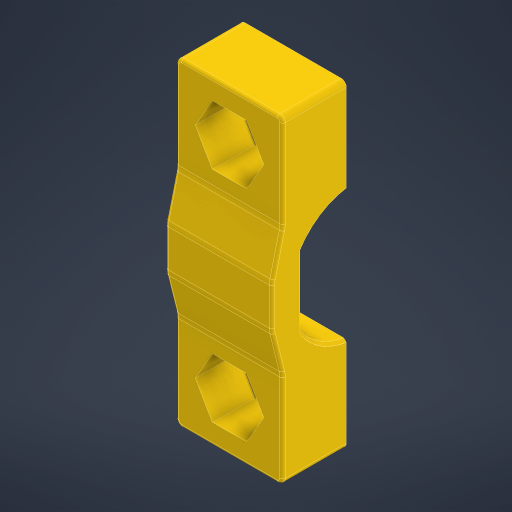
# Autodesk Inventor part: motor_C_clamp_nutt_motor_otoceny
Saved by Autodesk Inventor 2024 (Build 280153000, 153)
## iProperties
Created: 2023-08-14
Part Number: motor_C_clamp_nutt_motor_otoceny
Material: Všeobecné
Document SubType Name: Modeling
Designer: jaryj
Density: 1 g/cm^3
Appearance: Výchozí
Author: jaryj
Autodesk Inventor part; units mm, degrees
ref_plane "YZ Plane" through (0, 0, 0) normal (1, 0, 0) x (0, 1, 0)
ref_plane "XZ Plane" through (0, 0, 0) normal (0, 1, 0) x (-1, 0, 0)
ref_plane "XY Plane" through (0, 0, 0) normal (0, 0, 1) x (1, 0, 0)
sketch "Náčrt1" plane through (0, 0, 0) normal (0, 0, 1) x (1, 0, 0)
  line L0 (-5, 15) -> (5, 15)
  line L1 (5, 15) -> (5, -15)
  line L2 (5, -15) -> (-5, -15)
  line L3 (-5, -15) -> (-5, 15)
  line L4 (-5, 15) -> (5, -15) construction
  line L5 (5, 15) -> (-5, -15) construction
  circle A0 centre (0, 10.3125) radius 1.6
  circle A1 centre (0, -10.3125) radius 1.6
  line L6 (-5, 0) -> (5, 0)
  line L7 (0, 10.3125) -> (0, 15) construction
  line L8 (0, -10.3125) -> (0, -15) construction
  point P0 (0, 0)
  dimension "d0" = 30
  dimension "d1" = 10
  dimension "d2" = 3.2
  dimension "d42" = 20.625
  constraints: 18 end point, 6 midpoint, 2 centre point, 2 parallel, 2 vertical alignment, 1 equal radius, 1 horizontal, 1 perpendicular, 1 vertical, 1 other
  measures "d0" distance of L2.end L0.start
  measures "d1" distance of L0.start L0.end
  measures "d2" diameter of A0
  measures "d42" distance of L8.start L7.start
extrude "Vysunutí1" add sketch "Náčrt1" along normal blind 10
sketch "Náčrt2" plane through (5, -15, 0) normal (1, 0, 0) x (0, 0, -1)
  line L0 (0, 0) -> (0, 30) projected
  line L1 (0, 30) -> (-10, 30) projected
  line L2 (0, 0) -> (-10, 0) projected
  line L3 (-7, 0) -> (-7, 9.0003)
  line L4 (-7, 9.0003) -> (-8, 13)
  line L5 (-8, 17) -> (-7, 20.9997)
  line L6 (-7, 20.9997) -> (-7, 30)
  line L7 (-8, 13) -> (-8, 17)
  line L8 (-10, 0) -> (-10, 30) projected
  line L9 (-5, 11.6835) -> (-5, 18.3165)
  arc A0 (-5, 11.6835) -> (0, 9.0001) centre (0, 15) ccw
  arc A1 (0, 20.9999) -> (-5, 18.3165) centre (0, 15) ccw
  arc A2 (-5.125, 11.646) -> (0, 8.8751) centre (0, 15) ccw
  line L10 (-5.125, 11.646) -> (-5.125, 18.354)
  arc A3 (0, 21.1249) -> (-5.125, 18.354) centre (0, 15) ccw
  arc A4 (-7.5, 11.0001) -> (0, 6.5001) centre (0, 15) ccw construction
  line L11 (-7.5, 11.0001) -> (-7.5, 18.9999) construction
  arc A5 (0, 23.4999) -> (-7.5, 18.9999) centre (0, 15) ccw construction
  point P0 (0, 15)
  point P1 (0, 15)
  point P2 (0, 15)
  point P3 (-8, 15)
  point P4 (-10, 15)
  point P5 (-5, 15)
  point P6 (0, 8.8751)
  dimension "d17" = 3
  dimension "d18" = 3
  dimension "d19" = 2
  dimension "d47" = 6.633
  dimension "d49" = 5
  dimension "d51" = 5.9999
  dimension "d52" = 0.125
  dimension "d53" = 2.5
  dimension "d54" = 4
  constraints: 16 end point, 12 point on circle, 6 centre point, 5 midpoint, 2 coincident, 2 point on line, 1 equal length, 1 horizontal alignment, 1 perpendicular, 1 vertical, 11 other
  measures "d17" distance between parallel lines of L8 L3
  measures "d18" distance between parallel lines of L8 L6
  measures "d19" distance between parallel lines of L8 L7
  measures "d47" distance of L9.start L9.end
  measures "d49" distance of the line from the sketch origin of L9
  measures "d51" radius of A0
  measures "d52" radial gap between concentric circles of A0 A2
  measures "d53" radial gap between concentric circles of A0 A4
  measures "d54" distance of L4.end L5.start
extrude "Vysunutí2" cut sketch "Náčrt2" against normal through all contours A2 L10 A3 L0 A1 L9 A0 | L2 L8 L1 L6 L5 L7 L4 L3 | A0 L9 A1 L0
sketch "Náčrt7" plane through (0, 0, 0) normal (0, 0, -1) x (-1, 0, 0)
  line L0 (-5, 6.1249) -> (5, 6.1249) projected
  line L1 (5, 15) -> (5, 6.1249) projected
  line L2 (-5, 15) -> (5, 15) projected
  line L3 (-5, 6.1249) -> (-5, 15) projected
  circle A0 centre (0, 10.3125) radius 1.6 projected
  line L4 (5, -6.1249) -> (-5, -6.1249) projected
  line L5 (-5, -15) -> (-5, -6.1249) projected
  line L6 (5, -15) -> (-5, -15) projected
  line L7 (5, -6.1249) -> (5, -15) projected
  circle A1 centre (0, -10.3125) radius 1.6 projected
  line L8 (5, -3.354) -> (5, -6.1249) projected
  line L9 (-5, -3.354) -> (5, -3.354) projected
  line L10 (-5, -6.1249) -> (-5, -3.354) projected
  line L11 (5, -6.1249) -> (-5, -6.1249) projected
  line L12 (5, 6.1249) -> (5, 3.354) projected
  line L13 (-5, 6.1249) -> (5, 6.1249) projected
  line L14 (-5, 3.354) -> (-5, 6.1249) projected
  line L15 (-5, 3.354) -> (5, 3.354) projected
  point P0 (0, 0)
extrude "Vysunutí5" cut sketch "Náčrt7" against normal blind 1
fillet "Zaoblení1" radius 2 4 edges at (0, -2, 8) (0, 2, 8) (0, 5.9997, 7) (0, -5.9997, 7)
fillet "Zaoblení2" radius 0.25 20 edges at (0, -15, 7) (0, 15, 7) (5, -6.0016, 7.015) (5, -3.9999, 7.5) (5, -1.9982, 7.985) (5, 0, 8) (5, 1.9982, 7.985) (5, 3.9999, 7.5) (5, 6.0016, 7.015) (5, 10.623, 7) (5, -10.623, 7) (-5, -6.0016, 7.015) (-5, -3.9999, 7.5) (-5, -1.9982, 7.985) (-5, 0, 8) (-5, 1.9982, 7.985) (-5, 3.9999, 7.5) (-5, 6.0016, 7.015) (-5, 10.623, 7) (-5, -10.623, 7)
chamfer "Zkosení1" distance 0.25 angle 45 6 edges at (5, -5.1311, 3.3446) (5, 0, 5.125) (5, 5.1311, 3.3446) (-5, 5.1311, 3.3446) (-5, 0, 5.125) (-5, -5.1311, 3.3446)
fillet "Zaoblení3" radius 0.5 8 edges at (4.9268, -14.9268, 6.9268) (5, -15, 3.875) (-4.9268, -14.9268, 6.9268) (-5, -15, 3.875) (-4.9268, 14.9268, 6.9268) (-5, 15, 3.875) (4.9268, 14.9268, 6.9268) (5, 15, 3.875)
sketch "Náčrt4" plane through (-4.75, 6.2459, 7) normal (0, 0, 1) x (1, 0, 0)
  circle A0 centre (4.75, 4.0666) radius 1.6 projected
  point P0 (4.75, -6.2459)
  constraints: 1 coincident
sketch "Náčrt5" plane through (-4.75, -6.2459, 7) normal (0, 0, 1) x (1, 0, 0)
  circle A0 centre (4.75, -4.0666) radius 1.6 projected
  point P0 (4.75, 6.2459)
  constraints: 1 coincident
sketch "Náčrt6" plane through (-4.75, -6.2459, 7) normal (0, 0, 1) x (1, 0, 0)
  line L0 (1.5168, -4.0666) -> (3.1334, -1.2666)
  line L1 (3.1334, -1.2666) -> (6.3666, -1.2666)
  line L2 (6.3666, -1.2666) -> (7.9832, -4.0666)
  line L3 (7.9832, -4.0666) -> (6.3666, -6.8666)
  line L4 (6.3666, -6.8666) -> (3.1334, -6.8666)
  line L5 (3.1334, -6.8666) -> (1.5168, -4.0666)
  line L6 (1.5168, 16.5584) -> (3.1334, 19.3584)
  line L7 (3.1334, 19.3584) -> (6.3666, 19.3584)
  line L8 (6.3666, 19.3584) -> (7.9832, 16.5584)
  line L9 (7.9832, 16.5584) -> (6.3666, 13.7584)
  line L10 (6.3666, 13.7584) -> (3.1334, 13.7584)
  line L11 (3.1334, 13.7584) -> (1.5168, 16.5584)
  point P0 (4.75, 6.2459)
  point P1 (4.75, -4.0666)
  point P2 (4.75, 16.5584)
  point P3 (4.75, 16.5584)
  point P4 (4.75, 16.5584)
  point P5 (4.75, -4.0666)
  dimension "d43" = 5.6
  dimension "d44" = 5.6
  constraints: 24 end point, 2 coincident, 2 horizontal alignment, 26 other
  measures "d43" distance between parallel lines of L7 L10
  measures "d44" distance between parallel lines of L4 L1
extrude "Vysunutí4" cut sketch "Náčrt6" against normal blind 4
equation "\"d44\" = d43"
